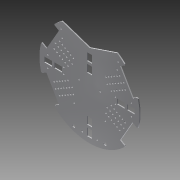
# Autodesk Inventor part: Bottom Plate
Saved by Autodesk Inventor 2015 (Build 190159000, 159)
## iProperties
Created: 2015-10-10
Part Number: Bottom Plate
Material: Polycarbonate, Clear
Document SubType Name: Modeling
Designer: James
Density: 1.2 g/cm^3
Appearance: Polycarbonate - Clear
Mass: 58.2697 g
Surface Area: 528.279 cm^2
Volume: 48.5581 cm^3
Author: James
Autodesk Inventor part; units mm, degrees
ref_plane "YZ Plane" through (0, 0, 0) normal (1, 0, 0) x (0, 1, 0)
ref_plane "XZ Plane" through (0, 0, 0) normal (0, 1, 0) x (-1, 0, 0)
ref_plane "XY Plane" through (0, 0, 0) normal (0, 0, 1) x (1, 0, 0)
sketch "Sketch1" plane through (0, 0, 0) normal (0, 1, 0) x (-1, 0, 0)
  line L0 (-73.6122, 42.5) -> (-86.1122, 20.8494)
  line L1 (-73.6122, 42.5) -> (-61.1122, 64.1506)
  line L2 (-73.6122, -42.5) -> (-61.1122, -64.1506)
  line L3 (-73.6122, -42.5) -> (-86.1122, -20.8494)
  line L4 (-86.1122, -20.8494) -> (-94.0858, -25.453)
  line L5 (-61.1122, -64.1506) -> (-69.0858, -68.7542)
  line L6 (-86.1122, 20.8494) -> (-94.0858, 25.453)
  line L7 (86.1122, 20.8494) -> (94.0858, 25.453)
  line L8 (73.6122, -42.5) -> (61.1122, -64.1506)
  line L9 (61.1122, -64.1506) -> (86.1122, -20.8494)
  line L10 (61.1122, -64.1506) -> (69.0858, -68.7542)
  line L11 (86.1122, -20.8494) -> (94.0858, -25.453)
  line L12 (-73.6122, -42.5) -> (-67.3622, -53.3253)
  line L13 (-73.6122, 42.5) -> (-79.8622, 31.6747)
  circle A0 centre (-68.0696, 39.3) radius 1.65
  circle A1 centre (-62.5703, 36.125) radius 1.65
  circle A2 centre (-57.0711, 32.95) radius 1.65
  circle A3 centre (-51.5718, 29.775) radius 1.65
  circle A4 centre (-46.0726, 26.6) radius 1.65
  circle A5 centre (-40.5733, 23.425) radius 1.65
  circle A6 centre (-35.074, 20.25) radius 1.65
  line L14 (-73.6122, 42.5) -> (-68.1872, 51.8964)
  circle A7 centre (-59.9599, 47.1464) radius 1.7
  circle A8 centre (-54.4607, 43.9714) radius 1.7
  circle A9 centre (-48.9614, 40.7964) radius 1.7
  circle A10 centre (-43.4621, 37.6214) radius 1.7
  circle A11 centre (-37.9629, 34.4464) radius 1.7
  circle A12 centre (-32.4636, 31.2714) radius 1.7
  circle A13 centre (-70.8099, 28.3536) radius 1.7
  circle A14 centre (-65.3107, 25.1786) radius 1.7
  circle A15 centre (-59.8114, 22.0036) radius 1.7
  circle A16 centre (-54.3121, 18.8286) radius 1.7
  circle A17 centre (-48.8129, 15.6536) radius 1.7
  circle A18 centre (-43.3136, 12.4786) radius 1.7
  circle A19 centre (68.0696, 39.3) radius 1.65
  circle A20 centre (62.5703, 36.125) radius 1.65
  circle A21 centre (57.0711, 32.95) radius 1.65
  circle A22 centre (51.5718, 29.775) radius 1.65
  circle A23 centre (46.0726, 26.6) radius 1.65
  circle A24 centre (40.5733, 23.425) radius 1.65
  circle A25 centre (35.074, 20.25) radius 1.65
  circle A26 centre (70.8099, 28.3536) radius 1.7
  circle A27 centre (65.3107, 25.1786) radius 1.7
  circle A28 centre (59.8114, 22.0036) radius 1.7
  circle A29 centre (54.3121, 18.8286) radius 1.7
  circle A30 centre (48.8129, 15.6536) radius 1.7
  circle A31 centre (43.3136, 12.4786) radius 1.7
  circle A32 centre (59.9599, 47.1464) radius 1.7
  circle A33 centre (54.4607, 43.9714) radius 1.7
  circle A34 centre (48.9614, 40.7964) radius 1.7
  circle A35 centre (43.4621, 37.6214) radius 1.7
  circle A36 centre (37.9629, 34.4464) radius 1.7
  circle A37 centre (32.4636, 31.2714) radius 1.7
  circle A38 centre (68.0696, -39.3) radius 1.65
  circle A39 centre (62.5703, -36.125) radius 1.65
  circle A40 centre (57.0711, -32.95) radius 1.65
  circle A41 centre (51.5718, -29.775) radius 1.65
  circle A42 centre (46.0726, -26.6) radius 1.65
  circle A43 centre (40.5733, -23.425) radius 1.65
  circle A44 centre (35.074, -20.25) radius 1.65
  circle A45 centre (59.9599, -47.1464) radius 1.7
  circle A46 centre (54.4607, -43.9714) radius 1.7
  circle A47 centre (48.9614, -40.7964) radius 1.7
  circle A48 centre (43.4621, -37.6214) radius 1.7
  circle A49 centre (37.9629, -34.4464) radius 1.7
  circle A50 centre (32.4636, -31.2714) radius 1.7
  circle A51 centre (70.8099, -28.3536) radius 1.7
  circle A52 centre (65.3107, -25.1786) radius 1.7
  circle A53 centre (59.8114, -22.0036) radius 1.7
  circle A54 centre (54.3121, -18.8286) radius 1.7
  circle A55 centre (48.8129, -15.6536) radius 1.7
  circle A56 centre (43.3136, -12.4786) radius 1.7
  circle A57 centre (-68.0696, -39.3) radius 1.65
  circle A58 centre (-62.5703, -36.125) radius 1.65
  circle A59 centre (-57.0711, -32.95) radius 1.65
  circle A60 centre (-51.5718, -29.775) radius 1.65
  circle A61 centre (-46.0726, -26.6) radius 1.65
  circle A62 centre (-40.5733, -23.425) radius 1.65
  circle A63 centre (-35.074, -20.25) radius 1.65
  circle A64 centre (-70.8099, -28.3536) radius 1.7
  circle A65 centre (-65.3107, -25.1786) radius 1.7
  circle A66 centre (-59.8114, -22.0036) radius 1.7
  circle A67 centre (-54.3121, -18.8286) radius 1.7
  circle A68 centre (-48.8129, -15.6536) radius 1.7
  circle A69 centre (-43.3136, -12.4786) radius 1.7
  circle A70 centre (-59.9599, -47.1464) radius 1.7
  circle A71 centre (-54.4607, -43.9714) radius 1.7
  circle A72 centre (-48.9614, -40.7964) radius 1.7
  circle A73 centre (-43.4621, -37.6214) radius 1.7
  circle A74 centre (-37.9629, -34.4464) radius 1.7
  circle A75 centre (-32.4636, -31.2714) radius 1.7
  arc A76 (-97.0264, 24.205) -> (-97.0264, -24.205) centre (0, 0) ccw
  arc A77 (-69.4754, -71.9248) -> (69.4754, -71.9248) centre (0, 0) ccw
  arc A78 (97.0264, -24.205) -> (97.0264, 24.205) centre (0, 0) ccw
  arc A79 (97.0264, 24.205) -> (94.0858, 25.453) centre (95.0858, 23.7209) ccw
  arc A80 (94.0858, -25.453) -> (97.0264, -24.205) centre (95.0858, -23.7209) ccw
  arc A81 (69.4754, -71.9248) -> (69.0858, -68.7542) centre (68.0858, -70.4863) ccw
  arc A82 (-97.0264, -24.205) -> (-94.0858, -25.453) centre (-95.0858, -23.7209) ccw
  arc A83 (-69.0858, -68.7542) -> (-69.4754, -71.9248) centre (-68.0858, -70.4863) ccw
  arc A84 (-94.0858, 25.453) -> (-97.0264, 24.205) centre (-95.0858, 23.7209) ccw
  line L15 (0, 55) -> (-5, 55)
  line L16 (-5, 55) -> (-5, 40)
  line L17 (-5, 40) -> (0, 40)
  line L18 (0, 40) -> (5, 40)
  line L19 (5, 40) -> (5, 55)
  line L20 (5, 55) -> (0, 55)
  line L21 (0, 35) -> (5, 35)
  line L22 (5, 35) -> (5, 20)
  line L23 (5, 20) -> (-5, 20)
  line L24 (-5, 20) -> (-5, 35)
  line L25 (-5, 35) -> (0, 35)
  line L26 (-90, 0) -> (-90, 5)
  line L27 (-90, 5) -> (-75, 5)
  line L28 (-75, 5) -> (-75, -5)
  line L29 (-75, -5) -> (-90, -5)
  line L30 (-90, -5) -> (-90, 0)
  line L31 (-70, 0) -> (-70, 5)
  line L32 (-70, 5) -> (-55, 5)
  line L33 (-55, 5) -> (-55, -5)
  line L34 (-55, -5) -> (-70, -5)
  line L35 (-70, -5) -> (-70, 0)
  line L36 (90, 0) -> (90, 5)
  line L37 (90, 5) -> (75, 5)
  line L38 (75, 5) -> (75, -5)
  line L39 (75, -5) -> (90, -5)
  line L40 (90, -5) -> (90, 0)
  line L41 (70, 0) -> (70, 5)
  line L42 (70, 5) -> (55, 5)
  line L43 (55, 5) -> (55, -5)
  line L44 (55, -5) -> (70, -5)
  line L45 (70, -5) -> (70, 0)
  line L46 (0, -90) -> (5, -90)
  line L47 (5, -90) -> (5, -75)
  line L48 (5, -75) -> (-5, -75)
  line L49 (-5, -75) -> (-5, -90)
  line L50 (-5, -90) -> (0, -90)
  line L51 (0, -70) -> (5, -70)
  line L52 (5, -70) -> (5, -55)
  line L53 (5, -55) -> (-5, -55)
  line L54 (-5, -55) -> (-5, -70)
  line L55 (-5, -70) -> (0, -70)
  circle A85 centre (-54.9519, 54.8205) radius 1.65
  circle A86 centre (54.9519, 54.8205) radius 1.65
  circle A87 centre (-20.9808, 0) radius 1.65
  circle A88 centre (20.9808, 0) radius 1.65
  circle A89 centre (-14.6505, -86.7861) radius 1.65
  circle A90 centre (14.6505, -86.7861) radius 1.65
  circle A91 centre (51.6401, 6.133) radius 1.65
  circle A92 centre (51.6401, -6.133) radius 1.65
  circle A93 centre (83.498, 11.6868) radius 1.65
  circle A94 centre (83.498, -11.6868) radius 1.65
  circle A95 centre (-51.6401, 6.133) radius 1.65
  circle A96 centre (-51.6401, -6.133) radius 1.65
  circle A97 centre (-83.498, 11.6868) radius 1.65
  circle A98 centre (-83.498, -11.6868) radius 1.65
  line L56 (90, 5) -> (75, 5)
  line L57 (75, 5) -> (75, -5)
  line L58 (75, -5) -> (90, -5)
  line L59 (90, -5) -> (90, 5)
  line L60 (70, 5) -> (55, 5)
  line L61 (55, 5) -> (55, -5)
  line L62 (55, -5) -> (70, -5)
  line L63 (70, -5) -> (70, 5)
  line L64 (5, 55) -> (-5, 55)
  line L65 (-5, 55) -> (-5, 40)
  line L66 (-5, 40) -> (5, 40)
  line L67 (5, 40) -> (5, 55)
  line L68 (5, 35) -> (-5, 35)
  line L69 (-5, 35) -> (-5, 20)
  line L70 (-5, 20) -> (5, 20)
  line L71 (5, 20) -> (5, 35)
  line L72 (5, -55) -> (-5, -55)
  line L73 (-5, -55) -> (-5, -70)
  line L74 (-5, -70) -> (5, -70)
  line L75 (5, -70) -> (5, -55)
  line L76 (5, -75) -> (-5, -75)
  line L77 (-5, -75) -> (-5, -90)
  line L78 (-5, -90) -> (5, -90)
  line L79 (5, -90) -> (5, -75)
  line L80 (-55, 5) -> (-70, 5)
  line L81 (-70, 5) -> (-70, -5)
  line L82 (-70, -5) -> (-55, -5)
  line L83 (-55, -5) -> (-55, 5)
  line L84 (-75, 5) -> (-90, 5)
  line L85 (-90, 5) -> (-90, -5)
  line L86 (-90, -5) -> (-75, -5)
  line L87 (-75, -5) -> (-75, 5)
  arc A99 (97.0264, -24.205) -> (97.0264, 24.205) centre (0, 0) ccw
  arc A100 (-69.4754, -71.9248) -> (69.4754, -71.9248) centre (0, 0) ccw
  arc A101 (-97.0264, 24.205) -> (-97.0264, -24.205) centre (0, 0) ccw
  arc A102 (97.0264, 24.205) -> (94.0858, 25.453) centre (95.0858, 23.7209) ccw
  arc A103 (94.0858, -25.453) -> (97.0264, -24.205) centre (95.0858, -23.7209) ccw
  arc A104 (69.4754, -71.9248) -> (69.0858, -68.7542) centre (68.0858, -70.4863) ccw
  arc A105 (-69.0858, -68.7542) -> (-69.4754, -71.9248) centre (-68.0858, -70.4863) ccw
  arc A106 (-97.0264, -24.205) -> (-94.0858, -25.453) centre (-95.0858, -23.7209) ccw
  arc A107 (-94.0858, 25.453) -> (-97.0264, 24.205) centre (-95.0858, 23.7209) ccw
  line L88 (-61.1122, 64.1506) -> (-86.1122, 20.8494)
  line L89 (-86.1122, 20.8494) -> (-94.0858, 25.453)
  line L90 (86.1122, 20.8494) -> (94.0858, 25.453)
  line L91 (86.1122, -20.8494) -> (94.0858, -25.453)
  line L92 (86.1122, -20.8494) -> (61.1122, -64.1506)
  line L93 (61.1122, -64.1506) -> (69.0858, -68.7542)
  line L94 (-69.0858, -68.7542) -> (-61.1122, -64.1506)
  line L95 (-61.1122, -64.1506) -> (-86.1122, -20.8494)
  line L96 (-86.1122, -20.8494) -> (-94.0858, -25.453)
  line L97 (-61.1122, 64.1506) -> (-69.0858, 68.7542)
  line L98 (61.1122, 64.1506) -> (69.0858, 68.7542)
  arc A108 (69.0858, 68.7542) -> (69.4754, 71.9248) centre (68.0858, 70.4863) ccw
  arc A109 (-69.4754, 71.9248) -> (-69.0858, 68.7542) centre (-68.0858, 70.4863) ccw
  arc A110 (-55.823, 82.9686) -> (-69.4754, 71.9248) centre (0, 0) ccw
  arc A111 (69.4754, 71.9248) -> (55.823, 82.9686) centre (0, 0) ccw
  line L99 (-54.0684, 83.2047) -> (0, 65)
  line L100 (0, 65) -> (54.0684, 83.2047)
  arc A112 (-54.0684, 83.2047) -> (-55.823, 82.9686) centre (-54.7066, 81.3092) ccw
  arc A113 (55.823, 82.9686) -> (54.0684, 83.2047) centre (54.7066, 81.3092) ccw
  arc A114 (55.823, 82.9686) -> (54.0684, 83.2047) centre (54.7066, 81.3092) ccw
  circle A115 centre (-31.1833, -85.6755) radius 3
  circle A116 centre (31.1833, -85.6755) radius 3
  line L101 (61.1122, 64.1506) -> (86.1122, 20.8494)
  line L102 (86.1122, 20.8494) -> (94.0858, 25.453)
  line L103 (94.0858, -25.453) -> (86.1122, -20.8494)
  line L104 (86.1122, -20.8494) -> (61.1122, -64.1506)
  line L105 (61.1122, -64.1506) -> (69.0858, -68.7542)
  line L106 (-69.0858, -68.7542) -> (-61.1122, -64.1506)
  line L107 (-61.1122, -64.1506) -> (-86.1122, -20.8494)
  line L108 (-86.1122, -20.8494) -> (-94.0858, -25.453)
  line L109 (-94.0858, 25.453) -> (-86.1122, 20.8494)
  line L110 (-86.1122, 20.8494) -> (-61.1122, 64.1506)
  line L111 (-61.1122, 64.1506) -> (-69.0858, 68.7542)
  line L112 (-54.0684, 83.2047) -> (0, 65)
  line L113 (0, 65) -> (54.0684, 83.2047)
  arc A117 (-55.823, 82.9686) -> (-69.0858, 72.299) centre (0, 0) ccw
  arc A118 (69.4754, 71.9248) -> (55.823, 82.9686) centre (0, 0) ccw
  arc A119 (97.0264, -24.205) -> (97.0264, 24.205) centre (0, 0) ccw
  arc A120 (-69.4754, -71.9248) -> (69.4754, -71.9248) centre (0, 0) ccw
  arc A121 (-97.0264, 24.205) -> (-97.0264, -24.205) centre (0, 0) ccw
  arc A122 (-69.4754, 71.9248) -> (-69.0858, 68.7542) centre (-68.0858, 70.4863) ccw
  arc A123 (-94.0858, 25.453) -> (-97.0264, 24.205) centre (-95.0858, 23.7209) ccw
  arc A124 (-97.0264, -24.205) -> (-94.0858, -25.453) centre (-95.0858, -23.7209) ccw
  arc A125 (-69.0858, -68.7542) -> (-69.4754, -71.9248) centre (-68.0858, -70.4863) ccw
  arc A126 (69.4754, -71.9248) -> (69.0858, -68.7542) centre (68.0858, -70.4863) ccw
  arc A127 (94.0858, -25.453) -> (97.0264, -24.205) centre (95.0858, -23.7209) ccw
  arc A128 (97.0264, 24.205) -> (94.0858, 25.453) centre (95.0858, 23.7209) ccw
  arc A129 (69.0858, 68.7542) -> (69.4754, 71.9248) centre (68.0858, 70.4863) ccw
  arc A130 (55.823, 82.9686) -> (54.0684, 83.2047) centre (54.7066, 81.3092) ccw
  arc A131 (-54.0684, 83.2047) -> (-55.823, 82.9686) centre (-54.7066, 81.3092) ccw
  arc A132 (-69.4754, 71.9248) -> (-69.0858, 68.7542) centre (-68.0858, 70.4863) ccw
  circle A133 centre (-31.1833, -45.6755) radius 1.65
  circle A134 centre (31.1833, -45.6755) radius 1.65
  circle A135 centre (-56.8952, 69.5753) radius 1.65
  circle A136 centre (56.8952, 69.5753) radius 1.65
  constraints: 228 end point, 137 centre point, 88 point on circle, 24 coincident, 16 parallel, 15 perpendicular, 13 collinear, 8 horizontal, 3 point on line, 3 tangent
extrude "Extrusion4" add sketch "Sketch1" along normal blind 2
body "Solid4"
